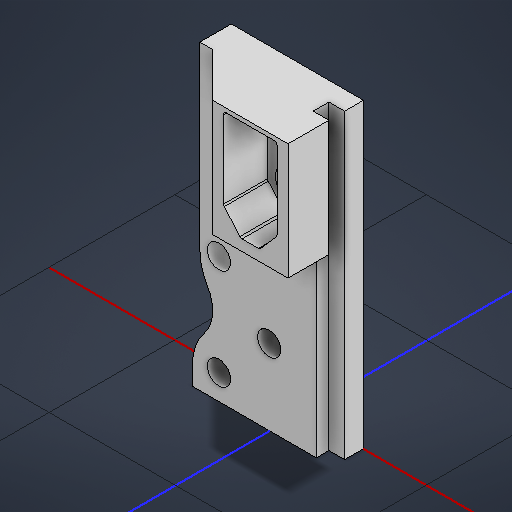
# Autodesk Inventor part: 000.011.001 - Основание
Saved by Autodesk Inventor 2025 (Build 290162000, 162)
## iProperties
Created: 2023-04-23
Part Number: 000.011.001 - Основание
Material: Типовые
Document SubType Name: Modeling
Designer: Иван Петров
Density: 1 g/cm^3
Appearance: По умолчанию
Author: Иван Петров
Autodesk Inventor part; units mm, degrees
ref_plane "YZ Plane" through (0, 0, 0) normal (1, 0, 0) x (0, 1, 0)
ref_plane "XZ Plane" through (0, 0, 0) normal (0, 1, 0) x (-1, 0, 0)
ref_plane "XY Plane" through (0, 0, 0) normal (0, 0, 1) x (1, 0, 0)
sketch "Эскиз1" plane through (0, 0, 0) normal (0, 0, 1) x (1, 0, 0)
  circle A0 centre (0, 0) radius 1.85 projected
  circle A1 centre (-8, -8) radius 1.85 projected
  circle A2 centre (-8, 8) radius 1.85 projected
  arc A3 (-12.1945, -4.6387) -> (-11.023, 3.351) centre (-16, 0) ccw projected
  line L0 (10, -14) -> (10, 42) projected
  line L1 (-12.1945, -4.6387) -> (-12.1945, -12)
  line L2 (-12.1945, -12) -> (10, -12)
  line L3 (-11.023, 3.351) -> (-11.023, 16)
  line L4 (-11.023, 16) -> (10, 16)
  point P0 (0, 0)
  dimension "d0" = 28
  dimension "d1" = 2
  constraints: 8 end point, 2 perpendicular, 2 point on line, 2 vertical
  measures "d0" distance between parallel lines of L2 L4
  measures "d1" distance from line of L0.start L2
extrude "Выдавливание1" add sketch "Эскиз1" along normal blind 5
fillet "Сопряжение1" radius 8.25 2 edges at (-12.1945, -4.6387, 2.5) (-11.023, 3.351, 2.5)
move faces "Перенос1" translate (1, 0, 0) faces at (-10.6884, -2.7905, 3.3333)
move faces "Перенос2" translate (0, 20, 0) faces at (2.9923, 16, 1.6667)
sketch "Эскиз2" plane through (0, 0, 5) normal (0, 0, 1) x (1, 0, 0)
  line L0 (8, 22.5746) -> (8, 34.9) projected
  arc A0 (8, 34.9) -> (7.8, 35.1) centre (7.8, 34.9) ccw projected
  line L1 (7.8, 35.1) -> (0.2, 35.1) projected
  arc A1 (0.2, 35.1) -> (0, 34.9) centre (0.2, 34.9) ccw projected
  line L2 (0, 34.9) -> (0, 22.5746) projected
  arc A2 (0, 22.5746) -> (0.0489, 22.4436) centre (0.2, 22.5746) ccw projected
  line L3 (0.0489, 22.4436) -> (2.5402, 19.569) projected
  line L4 (2.6913, 19.5) -> (5.3087, 19.5) projected
  arc A3 (2.5402, 19.569) -> (2.6913, 19.5) centre (2.6913, 19.7) ccw projected
  line L5 (5.4598, 19.569) -> (7.9511, 22.4436) projected
  arc A4 (5.3087, 19.5) -> (5.4598, 19.569) centre (5.3087, 19.7) ccw projected
  arc A5 (7.9511, 22.4436) -> (8, 22.5746) centre (7.8, 22.5746) ccw projected
  line L6 (10, -12) -> (10, 36) projected
  line L7 (10, 36) -> (-2, 36)
  line L8 (-2, 36) -> (-2, 17.5)
  line L9 (-2, 17.5) -> (10, 17.5)
  line L10 (10, 17.5) -> (10, 36)
  point P0 (0, 0)
  dimension "d11" = 2
  dimension "d12" = 2
  dimension "d13" = 2
  constraints: 8 end point, 2 parallel, 1 horizontal, 1 perpendicular
  measures "d11" distance between parallel lines of L6 L0
  measures "d12" distance between parallel lines of L8 L2
  measures "d13" distance between parallel lines of L4 L9
extrude "Выдавливание2" add sketch "Эскиз2" along normal blind 7
chamfer "Фаска1" distance 7 angle 45 1 edges at (-2, 26.75, 5)
sketch "Эскиз3" plane through (0, 0, 0) normal (0, 0, -1) x (-1, 0, 0)
  circle A0 centre (-4, 23.5) radius 3 projected
  circle A1 centre (-4, 31.1) radius 3 projected
  point P0 (0, 0)
extrude "Выдавливание3" cut sketch "Эскиз3" against normal blind 7
offset faces "Размер1" outward -0.25 faces at (2.7333, 35.1, 7.3333) (0.0006, 34.9149, 7.3333) (0, 26.6831, 7.3333) (8, 30.7915, 7.3333) (7.9978, 34.9298, 9.6667) (4.4362, 19.5, 7.3333) (7.1207, 21.4854, 7.3333) (5.365, 19.5081, 9.6667) (7.9845, 22.4973, 9.6667) (1.7097, 20.5272, 7.3333) (0.01, 22.5122, 9.6667) (2.6771, 19.5005, 7.3333)
sketch "Эскиз5" plane through (-11.023, 36, 0) normal (0, 1, 0) x (1, 0, 0)
  line L0 (21.023, 0) -> (21.023, -12) projected
  line L1 (21.023, -5.5) -> (18.523, -5.5)
  line L2 (18.523, -5.5) -> (18.523, -3)
  line L3 (18.523, -3) -> (21.023, -3)
  line L4 (21.023, -3) -> (21.023, -5.5)
  line L5 (21.023, 0) -> (0, 0) projected
  point P0 (11.023, 0)
  dimension "d26" = 2.5
  dimension "d27" = 2.5
  dimension "d28" = 3
  constraints: 8 end point, 2 parallel, 1 horizontal, 1 perpendicular, 1 point on line
  measures "d26" distance of L2.end L3.end
  measures "d27" distance of L1.end L2.end
  measures "d28" distance between parallel lines of L5 L3
extrude "Выдавливание5" cut sketch "Эскиз5" against normal through all
equation "\"d12\" = d11"
